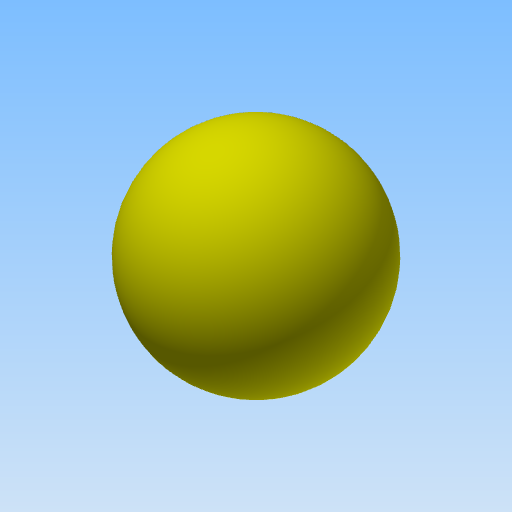
# Autodesk Inventor part: W 61704-2ZS_PART3
Saved by Autodesk Inventor 2020.2 (Build 242310000, 310)
## iProperties
Created: 2020-02-12
Part Number: W 61704-2ZS_PART3
Material: Allgemein
Catalog Web Link: www.cadenas.de
Description: -Deep groove ball bearings
Vendor: SKF
Document SubType Name: Modeling
Designer: psadmin
Manufacturer: SKF
Mass: 0.00209677 g
Surface Area: 0.0792229 cm^2
Volume: 0.00209677 cm^3
Density: 1 g/cm^3
Appearance: PSOLRGB-192-192-192
Category: PARTsolutions
Company: SKF
PSOL_IDENT_0: {$CADENAS_DATA\23d-libs\skf\bearings_units_and_housings\ball_bearings\deep_groove_ball_bearings\bb1_
PSOL_IDENT_1: 001_101.prj},201 {VTYP=3D},{NB=W 61704-2ZS_PART3},{LINA=W 61704-2ZS_PART3},{NN=BB1_001_101_PART3},{N
PSOL_IDENT_2: OPRJ=TRUE},{DATE=19.12.2019 14:34:47},{GEOMDATE=18.12.2019 13:53:11},{VERSION=},{LINEID=15490},{WBVA
PSOL_IDENT_3: R=},{WBNUMERIC=}  {NB=W 61704-2ZS_PART3},{LINA=W 61704-2ZS_PART3},{KT=DUMMY},{PRODUCTID=},{DESIGNATI
PSOL_IDENT_4: ON=W 61704-2ZS},{DD=20.000},{D=27.000},{B=4.000},{C=0.000},{DD1=22.36},{DD2=0.00},{D1=0.00},{D2=25.3
PSOL_IDENT_5: 0},{D3=0.000},{D4=0.000},{HH=MIN},{BB=0.000},{FF=0.00},{R0MAX=MIN},{R0=MIN},{R12=0.20},{PITCH=23.50}
PSOL_IDENT_6: ,{DW=1.588},{DDAMIN=21.500},{DDAMAX=22.000},{DDBMIN=MIN},{DDBMAX=MIN},{DBMIN=MIN},{DAMAX=26.000},{BB
PSOL_IDENT_7: AMIN=MIN},{CAMAX=MIN},{RAMAX=0.200},{LOAD1=0.585},{LOAD2=0.390},{LOAD3=0.017},{SPEED1=50000},{SPEED2=
PSOL_IDENT_8: 26000},{KR=0.015},{F0=8.700},{Z=18},{II=1},{MASS=0.006},{BEARING=W 61704-2ZS},{RING=},{HELP=1.218},{
PSOL_IDENT_9: HELP2=0.850},{DD1ALG=11.180},{YALG=11.180},{PITCH1=23.500},{DW1=1.588},{YALG1=12.282},{HALG1=1.218},
PSOL_IDENT_10: {SH=11.180},{CU=0.482},{DESIGN=dgbbw2z},{HALG=1.18},{B1=0},{SHIELDHELP=2}
NT: Deep groove ball bearings
NB: W 61704-2ZS_PART3
NBSYN: $DESIGNATION._PART3
LINA: W 61704-2ZS_PART3
SUPPLIER: SKF
ARTICLENO: W 61704-2ZS_PART3
BOMINFO: W 61704-2ZS_PART3
CREATOR: CADENAS GmbH
Title: W 61704-2ZS_PART3
Author: Cadenas PARTsolutions
Comments: Deep groove ball bearings
Autodesk Inventor part; units mm, degrees
ref_plane "YZ Plane" through (0, 0, 0) normal (1, 0, 0) x (0, 1, 0)
ref_plane "XZ Plane" through (0, 0, 0) normal (0, 1, 0) x (-1, 0, 0)
ref_plane "XY Plane" through (0, 0, 0) normal (0, 0, 1) x (1, 0, 0)
sketch "Sketch_6" plane through (0, 0, 0) normal (0, 0, 1) x (1, 0, 0)
  line L0 (2.794, 11.75) -> (1.206, 11.75)
  arc A0 (2.794, 11.75) -> (1.206, 11.75) centre (2, 11.75) ccw
  line L1 (2.794, 11.75) -> (1.206, 11.75)
  dimension "d0" = 360
  constraints: 4 end point, 2 point on circle, 1 centre point
revolve "Revolution1" add sketch "Sketch_6" angle 360 about axis through (2.794, 11.75, 0) along (1, 0, 0)
body "Solid1"
